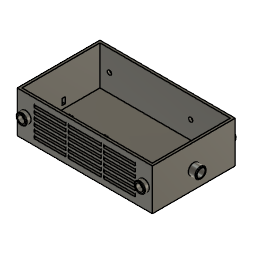
BoTech.StarClock.PowerSupplyBottom (Autodesk Fusion 360 design; units mm, degrees)
Autodesk Fusion 360 part; units mm, degrees
sketch "Skizze1" plane through (0, 0, 0) normal (0, 0, 1) x (1, 0, 0)
  line L0 (6, 66) -> (96, 66)
  line L1 (96, 66) -> (96, 14)
  line L2 (96, 14) -> (6, 14)
  line L3 (6, 14) -> (6, 66)
  line L4 (6, 14) -> (6, 4)
  line L5 (6, 66) -> (6, 68)
  line L6 (6, 66) -> (4, 66)
  line L7 (4, 66) -> (0, 66)
  line L8 (6, 4) -> (6, 0)
  line L9 (96, 66) -> (111, 66)
  line L10 (0, 0) -> (111, 0)
  line L11 (111, 0) -> (111, 68)
  line L12 (111, 68) -> (0, 68)
  line L13 (0, 68) -> (0, 0)
  line L14 (96, 14) -> (84, 14)
  line L15 (96, 66) -> (96, 55)
  line L16 (84, 14) -> (84, 55)
  line L17 (84, 55) -> (96, 55)
  circle A0 centre (90, 60) radius 2
  line L18 (90, 66) -> (90, 62)
  line L19 (96, 60) -> (92, 60)
  line L20 (111, 68) -> (111, 39)
  line L21 (111, 39) -> (111, 37)
  line L22 (111, 37) -> (121, 37)
  line L23 (111, 39) -> (121, 39)
  line L24 (121, 39) -> (121, 37)
  line L25 (111, 37) -> (111, 31)
  line L26 (111, 31) -> (121, 31)
  line L27 (121, 31) -> (121, 29)
  line L28 (121, 29) -> (111, 29)
  line L29 (111, 29) -> (111, 0)
  line L30 (-4, 32.6) -> (-4, 35.4)
  line L31 (-4, 35.4) -> (-4, 68)
  line L32 (-4, 32.6) -> (-4, 0)
  line L33 (0, 35.4) -> (-5, 35.4)
  line L34 (-5, 35.4) -> (-5, 37.4)
  line L35 (-5, 37.4) -> (0, 37.4)
  line L36 (0, 32.6) -> (-5, 32.6)
  line L37 (-5, 32.6) -> (-5, 30.6)
  line L38 (-5, 30.6) -> (0, 30.6)
  line L39 (2, 68) -> (2, 2)
  line L40 (2, 2) -> (109, 2)
  line L41 (109, 2) -> (109, 66)
  line L42 (96, 66) -> (109, 66)
  line L43 (109, 66) -> (111, 66)
  dimension "d1" = 90
  dimension "d2" = 52
  dimension "d3" = 10
  dimension "d4" = 2
  dimension "d6" = 2
  dimension "d7" = 4
  dimension "d8" = 4
  dimension "d9" = 15
  dimension "d10" = 111
  dimension "d11" = 68
  dimension "d12" = 12
  dimension "d13" = 11
  dimension "d14" = 4
  dimension "d15" = 4
  dimension "d16" = 4
  dimension "d22" = 29
  dimension "d23" = 2
  dimension "d24" = 10
  dimension "d26" = 6
  dimension "d27" = 10
  dimension "d28" = 2
  dimension "d29" = 29
  dimension "d30" = 2.8
  dimension "d31" = 32.6
  dimension "d32" = 32.6
  dimension "d33" = 5
  dimension "d34" = 2
  dimension "d35" = 5
  dimension "d36" = 2
  constraint horizontal L0
  constraint vertical L1
  constraint horizontal L2
  constraint vertical L3
  constraint perpendicular L2 L4
  constraint perpendicular L0 L5
  constraint perpendicular L5 L6
  constraint perpendicular L5 L7
  constraint parallel L4 L8
  constraint perpendicular L1 L9
  constraint horizontal L10
  constraint vertical L11
  constraint horizontal L12
  constraint vertical L13
  constraint coincident L10.start L13.end
  constraint perpendicular L1 L14
  constraint coincident L1 L15.end
  constraint perpendicular L14 L16
  constraint coincident L0 L18.start
  constraint perpendicular L0 L18
  constraint coincident L15 L19.start
  constraint perpendicular L1 L19
  constraint coincident L8.end L10
  constraint coincident L11 L20.end
  constraint perpendicular L12 L21
  constraint perpendicular L21 L22
  constraint perpendicular L11 L23
  constraint coincident L11 L25.end
  constraint perpendicular L25 L26
  constraint perpendicular L26 L27
  constraint coincident L11 L28.end
  constraint perpendicular L11 L28
  constraint perpendicular L10 L29
  constraint perpendicular L12 L30
  constraint parallel L30 L31
  constraint parallel L13 L32
  constraint coincident L13 L33.start
  constraint perpendicular L30 L33
  constraint perpendicular L33 L34
  constraint coincident L13 L35.end
  constraint perpendicular L13 L35
  constraint coincident L13 L36.start
  constraint perpendicular L32 L36
  constraint perpendicular L36 L37
  constraint coincident L13 L38.end
  constraint perpendicular L13 L38
  constraint coincident L12 L39.start
  constraint perpendicular L7 L39
  constraint perpendicular L39 L40
  constraint coincident L9 L41.end
  constraint perpendicular L9 L41
  measures "d1" distance of L0.start L0.end
  measures "d2" distance of L0.start L2.end
  measures "d3" distance of L2.end L4.end
  measures "d4" distance of L0.start L5.end
  measures "d6" distance of L0.start L6.end
  measures "d7" distance of L6.end L7.end
  measures "d8" distance of L4.end L8.end
  measures "d9" distance of L0.end L9.end
  measures "d10" distance of L10.start L10.end
  measures "d11" distance of L10.start L12.end
  measures "d12" distance of L1.end L14.end
  measures "d13" distance of L0.end L15.end
  measures "d14" diameter of A0
  measures "d15" distance of L18.start L18.end
  measures "d16" distance of L19.start L19.end
  measures "d22" distance of L11.end L20.end
  measures "d23" distance of L20.end L21.end
  measures "d24" distance of L21.end L22.end
  measures "d26" distance of L21.end L25.end
  measures "d27" distance of L25.end L26.end
  measures "d28" distance of L26.end L27.end
  measures "d29" distance of L28.end L10.end
  measures "d30" distance of L30.start L30.end
  measures "d31" distance of L30.end L31.end
  measures "d32" distance of L30.start L32.end
  measures "d33" distance of L33.start L33.end
  measures "d34" distance of L33.end L34.end
  measures "d35" distance of L36.start L36.end
  measures "d36" distance of L36.end L37.end
extrude "Extrusion1" add sketch "Skizze1" along normal blind 2 contours L0 L1 L2 L3 L15 L16 L17 A0 L18 L19 | L3 L4 L6 L7 L8 L39 L40 | L0 L1 L15 A0 L18 L19 | L1 L2 L4 L8 L9 L14 L15 L40 L41 L42 | A0 | L1 L2 L14 L16 L17
extrude "Extrusion2" add sketch "Skizze1" along normal blind 34 contours L0 L5 L9 L11 L12 L20 L42 L43 | L5 L6 L7 L12 L39 | L7 L12 L13 L39 | L7 L8 L10 L13 L39 L40 | L8 L9 L10 L11 L20 L21 L25 L29 L40 L41 L43
sketch "Skizze2" plane through (0, 68, 0) normal (0, 1, 0) x (-1, 0, 0)
  line L0 (-111, 0) -> (0, 0)
  line L1 (0, 0) -> (0, 34)
  line L2 (0, 34) -> (-111, 34)
  line L3 (-111, 34) -> (-111, 0)
  line L4 (0, 0) -> (0, 2)
  line L5 (0, 2) -> (-6, 2)
  line L6 (-6, 2) -> (-96, 2)
  line L7 (-9.75, 2) -> (-9.75, 15)
  circle A0 centre (-9.7507, 16.75) radius 1.75
  line L8 (-6, 2) -> (-6, 34)
  line L9 (-6, 16.7) -> (-8, 16.7)
  line L10 (-11.5, 16.7) -> (-74.75, 16.7)
  circle A1 centre (-76.5, 16.7) radius 1.75
  circle A2 centre (-76.5, 16.7) radius 3
  circle A3 centre (-9.7507, 16.75) radius 3
  circle A4 centre (-76.5, 16.7) radius 4.5
  circle A5 centre (-9.7507, 16.75) radius 4.5
  line L11 (-111, 17) -> (-104, 17)
  circle A6 centre (-104, 17) radius 1.75
  circle A7 centre (-76.5, 16.7) radius 1
  circle A8 centre (-104, 17) radius 3
  circle A9 centre (-104, 17) radius 4.5
  dimension "d43" = 2
  dimension "d44" = 6
  dimension "d45" = 90
  dimension "d46" = 13
  dimension "d47" = 3.5
  dimension "d48" = 2
  dimension "d49" = 63.25
  dimension "d50" = 3.5
  dimension "d51" = 6
  dimension "d52" = 6
  dimension "d55" = 9
  dimension "d56" = 9
  dimension "d61" = 7
  dimension "d62" = 3.5
  dimension "d150" = 2
  dimension "d151" = 6
  dimension "d152" = 9
  constraint coincident L0.end L1.start
  constraint perpendicular L0 L4
  constraint perpendicular L4 L5
  constraint perpendicular L4 L6
  constraint coincident L6 L7.start
  constraint perpendicular L6 L7
  constraint coincident L2 L8.end
  constraint perpendicular L2 L8
  constraint coincident L8 L9.start
  constraint perpendicular L8 L9
  constraint horizontal L10
  constraint coincident A0 L10.start
  constraint coincident L10.end A1
  constraint concentric A1 A2
  constraint concentric A0 A3
  constraint concentric A1 A4
  constraint concentric A0 A5
  constraint midpoint L3 L11.start
  constraint perpendicular L3 L11
  constraint coincident L11.end A6.centre
  constraint concentric A6 A8
  constraint concentric A8 A9
  measures "d43" distance of L0.end L4.end
  measures "d44" distance of L4.end L5.end
  measures "d45" distance of L5.end L6.end
  measures "d46" distance of L7.start L7.end
  measures "d47" diameter of A0
  measures "d48" distance of L9.start L9.end
  measures "d49" distance of L10.start L10.end
  measures "d50" diameter of A1
  measures "d51" diameter of A2
  measures "d52" diameter of A3
  measures "d55" diameter of A4
  measures "d56" diameter of A5
  measures "d61" distance of L11.start L11.end
  measures "d62" diameter of A6
  measures "d150" diameter of A7
  measures "d151" diameter of A8
  measures "d152" diameter of A9
extrude "Extrusion3" cut sketch "Skizze2" against normal blind 2 contours A0 | A1 | A6 | A7
extrude "Extrusion4" add sketch "Skizze2" along normal blind 3.75 contours L7 L8 L9 A3 A5 | L8 A5 | L8 L9 L10 A3 A5 | L7 L10 A3 A5 | A4 | A9
fillet "Abrundung1" radius 0.5 3 edges at (108.1955, 71.75, 15.3727) (80.6955, 71.75, 15.0727) (13.9462, 71.75, 15.1227)
sketch "Skizze3" plane through (0, 0, 0) normal (0, -1, 0) x (1, 0, 0)
  line L0 (0, 0) -> (111, 0)
  line L1 (111, 0) -> (111, 34)
  line L2 (111, 34) -> (0, 34)
  line L3 (0, 34) -> (0, 0)
  line L4 (0, 17) -> (7, 17)
  circle A0 centre (7, 17) radius 1.75
  line L5 (111, 17) -> (104, 17)
  circle A1 centre (104, 17) radius 1.75
  line L6 (14, 7) -> (97, 7)
  line L7 (97, 7) -> (97, 5)
  line L8 (97, 5) -> (14, 5)
  line L9 (14, 5) -> (14, 7)
  line L10 (97, 9.4) -> (14, 9.4)
  line L11 (14, 9.4) -> (14, 11.4)
  line L12 (97, 11.4) -> (97, 9.4)
  line L13 (14, 11.4) -> (97, 11.4)
  line L14 (97, 13.8) -> (14, 13.8)
  line L15 (14, 13.8) -> (14, 15.8)
  line L16 (97, 15.8) -> (97, 13.8)
  line L17 (14, 15.8) -> (97, 15.8)
  line L18 (97, 18.2) -> (14, 18.2)
  line L19 (14, 18.2) -> (14, 20.2)
  line L20 (97, 20.2) -> (97, 18.2)
  line L21 (14, 20.2) -> (97, 20.2)
  line L22 (97, 22.6) -> (14, 22.6)
  line L23 (14, 22.6) -> (14, 24.6)
  line L24 (97, 24.6) -> (97, 22.6)
  line L25 (14, 24.6) -> (97, 24.6)
  line L26 (97, 27) -> (14, 27)
  line L27 (14, 27) -> (14, 29)
  line L28 (97, 29) -> (97, 27)
  line L29 (14, 29) -> (97, 29)
  circle A2 centre (7, 17) radius 3
  circle A3 centre (7, 17) radius 4.5
  circle A4 centre (104, 17) radius 3
  circle A5 centre (104, 17) radius 4.5
  line L30 (14, 0) -> (12, 0)
  line L31 (12, 0) -> (12, 34)
  line L32 (12, 34) -> (14, 34)
  line L33 (14, 34) -> (14, 0)
  line L34 (97, 0) -> (99, 0)
  line L35 (99, 0) -> (99, 34)
  line L36 (99, 34) -> (97, 34)
  line L37 (97, 34) -> (97, 0)
  line L38 (14, 34) -> (40, 34)
  line L39 (40, 34) -> (42, 34)
  line L40 (42, 34) -> (42, 0)
  line L41 (42, 0) -> (40, 0)
  line L42 (40, 0) -> (40, 34)
  line L43 (97, 34) -> (71, 34)
  line L44 (71, 34) -> (69, 34)
  line L45 (69, 34) -> (69, 0)
  line L46 (69, 0) -> (71, 0)
  line L47 (71, 0) -> (71, 34)
  dimension "d68" = 7
  dimension "d69" = 3.5
  dimension "d70" = 7
  dimension "d71" = 3.5
  dimension "d76" = 0
  dimension "d77" = 22
  dimension "d136" = 6
  dimension "d137" = 9
  dimension "d138" = 6
  dimension "d139" = 9
  dimension "d140" = 2
  dimension "d141" = 2
  dimension "d142" = 26
  dimension "d143" = 2
  dimension "d144" = 26
  dimension "d145" = 2
  constraint midpoint L3 L4.start
  constraint perpendicular L3 L4
  constraint coincident L4.end A0.centre
  constraint midpoint L1 L5.start
  constraint perpendicular L1 L5
  constraint coincident L5.end A1.centre
  constraint horizontal L6
  constraint vertical L7
  constraint horizontal L8
  constraint vertical L9
  constraint concentric A0 A2
  constraint concentric A2 A3
  constraint concentric A1 A4
  constraint concentric A1 A5
  constraint horizontal L30
  constraint vertical L31
  constraint horizontal L32
  constraint vertical L33
  constraint coincident L2 L31.end
  constraint coincident L0 L30.start
  constraint horizontal L34
  constraint vertical L35
  constraint horizontal L36
  constraint vertical L37
  constraint coincident L2 L35.end
  constraint coincident L0 L34.start
  constraint coincident L2 L38.end
  constraint horizontal L39
  constraint vertical L40
  constraint horizontal L41
  constraint vertical L42
  constraint coincident L0 L40.end
  constraint coincident L2 L43.end
  constraint horizontal L44
  constraint vertical L45
  constraint horizontal L46
  constraint vertical L47
  constraint coincident L0 L45.end
  measures "d68" distance of L4.start L4.end
  measures "d69" diameter of A0
  measures "d70" distance of L5.start L5.end
  measures "d71" diameter of A1
  measures "d136" diameter of A2
  measures "d137" diameter of A3
  measures "d138" diameter of A4
  measures "d139" diameter of A5
  measures "d140" distance of L30.start L30.end
  measures "d141" distance of L34.start L34.end
  measures "d142" distance of L32.end L38.end
  measures "d143" distance of L38.end L39.end
  measures "d144" distance of L36.end L43.end
  measures "d145" distance of L43.end L44.end
extrude "Extrusion19" add sketch "Skizze3" along normal blind 3.75 contours A3 | A5
fillet "Abrundung5" radius 0.5 2 edges at (99.8045, -3.75, 15.3727) (2.8045, -3.75, 15.3727)
extrude "Extrusion5" cut sketch "Skizze3" against normal blind 2 contours L6 L8 L9 L33 L42 | L6 L8 L40 L42 | L26 L27 L29 L33 L42 | L6 L8 L40 L45 | L10 L11 L13 L33 L42 | L26 L29 L40 L42 | L6 L8 L45 L47 | L10 L13 L40 L42 | L26 L29 L40 L45 | L22 L23 L25 L33 L42 | L6 L7 L8 L37 L47 | L10 L13 L40 L45 | L14 L15 L17 L33 L42 | L26 L29 L45 L47 | L22 L25 L40 L42 | L10 L13 L45 L47 | L14 L17 L40 L42 | L26 L28 L29 L37 L47 | L22 L25 L40 L45 | L18 L19 L21 L33 L42 | L10 L12 L13 L37 L47 | L14 L17 L40 L45 | L22 L25 L45 L47 | L18 L21 L40 L42 | L14 L17 L45 L47 | L22 L24 L25 L37 L47 | L18 L21 L40 L45 | L14 L16 L17 L37 L47 | L18 L21 L45 L47 | L18 L20 L21 L37 L47 | A0 | A1
extrude "Extrusion18" add sketch "Skizze3" against normal blind 4 contours L0 L8 L40 L41 L42 | L6 L8 L40 L42 | L2 L29 L39 L40 L42 | L0 L8 L45 L46 L47 | L6 L10 L40 L42 | L26 L29 L40 L42 | L6 L8 L45 L47 | L10 L13 L40 L42 | L2 L29 L44 L45 L47 | L25 L26 L40 L42 | L6 L10 L45 L47 | L13 L14 L40 L42 | L26 L29 L45 L47 | L22 L25 L40 L42 | L10 L13 L45 L47 | L14 L17 L40 L42 | L25 L26 L45 L47 | L21 L22 L40 L42 | L13 L14 L45 L47 | L17 L18 L40 L42 | L22 L25 L45 L47 | L18 L21 L40 L42 | L14 L17 L45 L47 | L21 L22 L45 L47 | L17 L18 L45 L47 | L18 L21 L45 L47
fillet "Abrundung4" radius 2 4 edges at (41, 4, 34) (70, 4, 34) (41, 4, 34) (70, 4, 34)
sketch "Skizze7" plane through (14, 0, 0) normal (1, 0, 0) x (0, 1, 0)
  line L0 (0, 7) -> (0, 5)
  line L1 (0, 5) -> (2, 5)
  line L2 (2, 5) -> (2, 7)
  line L3 (2, 7) -> (0, 7)
  line L4 (0, 5) -> (2, 7)
  line L5 (0, 7) -> (2, 9.4)
  line L6 (0, 7) -> (0, 9.4)
  line L7 (0, 9.4) -> (2, 9.4)
  line L8 (2, 7) -> (2, 5)
  line L9 (0, 5) -> (2, 5)
  line L10 (0, 5) -> (0, 7)
  line L11 (2, 7) -> (2, 9.4)
  line L12 (0, 11.4) -> (0, 13.8)
  line L13 (0, 9.4) -> (2, 11.4)
  line L14 (2, 11.4) -> (2, 13.8)
  line L15 (2, 11.4) -> (2, 9.4)
  line L16 (0, 9.4) -> (2, 9.4)
  line L17 (2, 11.4) -> (0, 11.4)
  line L18 (0, 9.4) -> (2, 9.4)
  line L19 (0, 9.4) -> (0, 11.4)
  line L20 (2, 9.4) -> (2, 11.4)
  line L21 (0, 13.8) -> (2, 13.8)
  line L22 (0, 11.4) -> (2, 13.8)
  line L23 (0, 11.4) -> (0, 9.4)
  line L24 (0, 15.8) -> (0, 18.2)
  line L25 (0, 13.8) -> (2, 15.8)
  line L26 (2, 15.8) -> (2, 18.2)
  line L27 (2, 15.8) -> (2, 13.8)
  line L28 (0, 13.8) -> (2, 13.8)
  line L29 (2, 15.8) -> (0, 15.8)
  line L30 (0, 13.8) -> (2, 13.8)
  line L31 (0, 13.8) -> (0, 15.8)
  line L32 (2, 13.8) -> (2, 15.8)
  line L33 (0, 18.2) -> (2, 18.2)
  line L34 (0, 15.8) -> (2, 18.2)
  line L35 (0, 15.8) -> (0, 13.8)
  line L36 (0, 20.2) -> (0, 22.6)
  line L37 (0, 18.2) -> (2, 20.2)
  line L38 (2, 20.2) -> (2, 22.6)
  line L39 (2, 20.2) -> (2, 18.2)
  line L40 (0, 18.2) -> (2, 18.2)
  line L41 (2, 20.2) -> (0, 20.2)
  line L42 (0, 18.2) -> (2, 18.2)
  line L43 (0, 18.2) -> (0, 20.2)
  line L44 (2, 18.2) -> (2, 20.2)
  line L45 (0, 22.6) -> (2, 22.6)
  line L46 (0, 20.2) -> (2, 22.6)
  line L47 (0, 20.2) -> (0, 18.2)
  line L48 (0, 24.6) -> (0, 27)
  line L49 (0, 22.6) -> (2, 24.6)
  line L50 (2, 24.6) -> (2, 27)
  line L51 (2, 24.6) -> (2, 22.6)
  line L52 (0, 22.6) -> (2, 22.6)
  line L53 (2, 24.6) -> (0, 24.6)
  line L54 (0, 22.6) -> (2, 22.6)
  line L55 (0, 22.6) -> (0, 24.6)
  line L56 (2, 22.6) -> (2, 24.6)
  line L57 (0, 27) -> (2, 27)
  line L58 (0, 24.6) -> (2, 27)
  line L59 (0, 24.6) -> (0, 22.6)
  line L60 (0, 29) -> (0, 31.4)
  line L61 (0, 27) -> (2, 29)
  line L62 (2, 29) -> (2, 31.4)
  line L63 (2, 29) -> (2, 27)
  line L64 (0, 27) -> (2, 27)
  line L65 (2, 29) -> (0, 29)
  line L66 (0, 27) -> (2, 27)
  line L67 (0, 27) -> (0, 29)
  line L68 (2, 27) -> (2, 29)
  line L69 (0, 31.4) -> (2, 31.4)
  line L70 (0, 29) -> (2, 31.4)
  line L71 (0, 29) -> (0, 27)
  dimension "d108" = 0
  dimension "d109" = 22
  constraint coincident L0.end L1.start
  constraint coincident L2.end L3.start
  constraint coincident L0.start L3.end
  constraint perpendicular L3 L6
  constraint perpendicular L6 L7
  constraint coincident L1.end L2.start
extrude "Extrusion12" cut sketch "Skizze7" along normal blind 26 contours L3 L5 L11 | L14 L17 L22 | L26 L29 L34 | L38 L41 L46 | L50 L53 L58 | L62 L65 L70
extrude "Extrusion13" add sketch "Skizze7" along normal blind 26 contours L1 L2 L4 L8 L9 | L7 L13 L15 L16 L18 L20 | L21 L25 L27 L28 L30 L32 | L33 L37 L39 L40 L42 L44 | L45 L49 L51 L52 L54 L56 | L57 L61 L63 L64 L66 L68
extrude "Extrusion14" cut sketch "Skizze7" along normal blind 27 from surface at 28 contours L3 L5 L11 | L14 L17 L22 | L26 L29 L34 | L38 L41 L46 | L50 L53 L58 | L62 L65 L70
extrude "Extrusion15" add sketch "Skizze7" along normal blind 27 from surface at 28 contours L1 L2 L4 L8 L9 | L7 L13 L15 L16 L18 L20 | L21 L25 L27 L28 L30 L32 | L33 L37 L39 L40 L42 L44 | L45 L49 L51 L52 L54 L56 | L57 L61 L63 L64 L66 L68
extrude "Extrusion16" cut sketch "Skizze7" along normal blind 26 from surface at 57 contours L3 L5 L11 | L14 L17 L22 | L26 L29 L34 | L38 L41 L46 | L50 L53 L58 | L62 L65 L70
extrude "Extrusion17" add sketch "Skizze7" along normal blind 27 from surface at 57 contours L1 L2 L4 L8 L9 | L7 L13 L15 L16 L18 L20 | L21 L25 L27 L28 L30 L32 | L33 L37 L39 L40 L42 L44 | L45 L49 L51 L52 L54 L56 | L57 L61 L63 L64 L66 L68
sketch "Skizze4" plane through (111, 0, 0) normal (1, 0, 0) x (0, 1, 0)
  line L0 (0, 0) -> (68, 0)
  line L1 (68, 0) -> (68, 34)
  line L2 (68, 34) -> (0, 34)
  line L3 (0, 34) -> (0, 0)
  circle A0 centre (34, 15) radius 3.375
  circle A1 centre (34, 15) radius 4.5
  dimension "d90" = 6.75
  dimension "d91" = 9
  constraint concentric A0 A1
  measures "d90" diameter of A0
  measures "d91" diameter of A1
extrude "Extrusion8" cut sketch "Skizze4" against normal blind 2 contours A0
extrude "Extrusion9" add sketch "Skizze4" along normal blind 6 contours A1
sketch "Skizze6" plane through (0, 0, 0) normal (-1, 0, 0) x (0, -1, 0)
  line L0 (-68, 0) -> (0, 0)
  line L1 (0, 0) -> (0, 34)
  line L2 (0, 34) -> (-68, 34)
  line L3 (-68, 34) -> (-68, 0)
  line L4 (-35, 5) -> (-35, 10)
  line L5 (-37.5, 10) -> (-37.5, 5)
  line L6 (-37.5, 5) -> (-35, 5)
  line L7 (-35, 10) -> (-37.5, 10)
  line L8 (-39.5, 12) -> (-33, 12)
  line L9 (-33, 12) -> (-33, 3)
  line L10 (-33, 3) -> (-39.5, 3)
  line L11 (-39.5, 3) -> (-39.5, 12)
  dimension "d96" = 5
  dimension "d97" = 2.5
  constraint horizontal L8
  constraint vertical L9
  constraint horizontal L10
  constraint vertical L11
  measures "d96" distance of L5.start L5.end
  measures "d97" distance of L4.end L5.start
extrude "Extrusion10" cut sketch "Skizze6" against normal blind 2 contours L4 L5 L6 L7
extrude "Extrusion11" add sketch "Skizze6" along normal blind 3 contours L8 L9 L10 L11
fillet "Abrundung2" radius 0.5 4 edges at (-1.5, 33, 12) (-1.5, 39.5, 12) (-1.5, 33, 3) (-1.5, 39.5, 3)
fillet "Abrundung3" radius 0.5 1 edges at (117, 29.8045, 13.3727)
